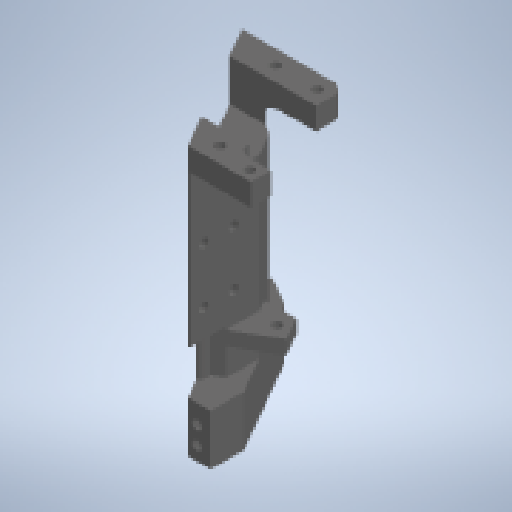
# Autodesk Inventor part: base_plate_towheel_front_left
Saved by Autodesk Inventor 2024.1 (Build 281209000, 209)
## iProperties
Created: 2025-02-03
Part Number: base_plate_towheel_front_left
Material: 一般
Document SubType Name: モデリング
Designer: hibik
Density: 1 g/cm^3
Appearance: 既定
Sheet Metal Rule: Default_mm
Author: hibik
Autodesk Inventor part; units mm, degrees
ref_plane "YZ Plane" through (0, 0, 0) normal (1, 0, 0) x (0, 1, 0)
ref_plane "XZ Plane" through (0, 0, 0) normal (0, 1, 0) x (-1, 0, 0)
ref_plane "XY Plane" through (0, 0, 0) normal (0, 0, 1) x (1, 0, 0)
sketch "スケッチ1" plane through (0, 0, 0) normal (0, 1, 0) x (-1, 0, 0)
  line L0 (75, 0) -> (105, -51.9615)
  line L1 (-75, 0) -> (-105, -51.9615)
  line L2 (0, -220.136) -> (0, 47.7586) projected
  line L3 (147, 0) -> (-147, 0) projected
  line L4 (37.5, -27) -> (-37.5, -27)
  line L5 (105, -51.9615) -> (30, -181.8653)
  line L6 (30, -181.8653) -> (-30, -181.8653)
  line L7 (-30, -181.8653) -> (-105, -51.9615)
  line L8 (75, 0) -> (-75, 0)
  line L9 (-25.3673, -135.8894) -> (-62.8673, -70.9375)
  line L10 (25.3673, -135.8894) -> (62.8673, -70.9375)
  line L11 (-37.5, -27) -> (-27.5, -27)
  line L12 (-27.5, -27) -> (-27.5, -39)
  line L13 (-27.5, -39) -> (-37.5, -39)
  line L14 (-37.5, -39) -> (-37.5, -27)
  line L15 (37.5, -27) -> (27.5, -27)
  line L16 (27.5, -27) -> (27.5, -39)
  line L17 (27.5, -39) -> (37.5, -39)
  line L18 (37.5, -39) -> (37.5, -27)
  line L19 (0, -77.9423) -> (44.1173, -103.4134) construction
  line L20 (0, -77.9423) -> (-44.1173, -103.4134) construction
  line L21 (-44.1173, -103.4134) -> (-67.5, -116.9134) construction
  line L22 (-57.8673, -79.5977) -> (-47.475, -73.5977)
  line L23 (-52.475, -64.9375) -> (-62.8673, -70.9375)
  line L24 (-62.8673, -70.9375) -> (-57.8673, -79.5977)
  line L25 (-47.475, -73.5977) -> (-52.475, -64.9375)
  line L26 (-25.3673, -135.8894) -> (-30.3673, -127.2291)
  line L27 (-19.975, -121.2291) -> (-14.975, -129.8894)
  line L28 (-14.975, -129.8894) -> (-25.3673, -135.8894)
  line L29 (-30.3673, -127.2291) -> (-19.975, -121.2291)
  line L30 (30.3673, -127.2291) -> (19.975, -121.2291)
  line L31 (14.975, -129.8894) -> (25.3673, -135.8894)
  line L32 (25.3673, -135.8894) -> (30.3673, -127.2291)
  line L33 (19.975, -121.2291) -> (14.975, -129.8894)
  line L34 (62.8673, -70.9375) -> (57.8673, -79.5977)
  line L35 (47.475, -73.5977) -> (52.475, -64.9375)
  line L36 (52.475, -64.9375) -> (62.8673, -70.9375)
  line L37 (57.8673, -79.5977) -> (47.475, -73.5977)
  line L38 (62.8673, -70.9375) -> (37.5, -27)
  line L39 (-37.5, -27) -> (-62.8673, -70.9375)
  line L40 (-25.3673, -135.8894) -> (25.3673, -135.8894)
  line L41 (-27.5, -39) -> (-47.475, -73.5977)
  point P0 (0, 0)
  point P1 (0, 0)
  point P2 (0, -27)
  dimension "d1" = 150
  dimension "d2" = 60
  dimension "d3" = 60
  dimension "d4" = 27
  dimension "d5" = 75
  dimension "d6" = 60
  dimension "d7" = 27
  dimension "d8" = 10
  dimension "d9" = 12
  dimension "d10" = 10
  dimension "d11" = 12
  dimension "d14" = 360
  constraints: 80 end point, 6 equal length, 6 parallel, 4 horizontal, 4 midpoint, 3 coincident, 3 perpendicular, 2 symmetric about line, 1 collinear, 1 horizontal alignment, 1 point on line, 1 vertical alignment, 50 other
  measures "d1" distance of L1.start L0.start
  measures "d2" angle of L3 L0
  measures "d3" angle of L1 L3
  measures "d4" distance between parallel lines of L3 L4
  measures "d5" distance of L4.start L4.end
  measures "d6" distance of L5.end L6.end
  measures "d7" distance between parallel lines of L7 L9
  measures "d8" distance of L12.end L13.end
  measures "d9" distance of L11.end L12.end
  measures "d10" distance of L17.end L16.end
  measures "d11" distance of L16.end L15.end
extrude "押し出し1" add sketch "スケッチ1" along normal blind 18.3 contours L12 L13 L14 L4 | L14 L13 L41 L25 L23 L39 | L23 L25 L22 L9
sketch "スケッチ2" plane through (27.5, 0, -27) normal (0, 0, 1) x (1, 0, 0)
  circle A0 centre (5, 11.5) radius 1.6 projected
  circle A1 centre (5, 5) radius 1.6 projected
  point P0 (-27.5, 0)
sketch "スケッチ3" plane through (27.5, 0, -27) normal (0, 0, 1) x (1, 0, 0)
  circle A0 centre (5, 11.5) radius 1.6 projected
  circle A1 centre (5, 5) radius 1.6 projected
  line L0 (8.2909, 11.5) -> (6.6454, 8.65)
  line L1 (6.6454, 8.65) -> (3.3546, 8.65)
  line L2 (3.3546, 8.65) -> (1.7091, 11.5)
  line L3 (1.7091, 11.5) -> (3.3546, 14.35)
  line L4 (3.3546, 14.35) -> (6.6454, 14.35)
  line L5 (6.6454, 14.35) -> (8.2909, 11.5)
  line L6 (6.6454, 7.85) -> (8.2909, 5)
  line L7 (8.2909, 5) -> (6.6454, 2.15)
  line L8 (6.6454, 2.15) -> (3.3546, 2.15)
  line L9 (3.3546, 2.15) -> (1.7091, 5)
  line L10 (1.7091, 5) -> (3.3546, 7.85)
  line L11 (3.3546, 7.85) -> (6.6454, 7.85)
  point P0 (-27.5, 0)
  dimension "d19" = 5.7
  constraints: 24 end point, 2 coincident, 2 horizontal, 1 parallel, 26 other
  measures "d19" distance from line of L0.end L4
extrude "押し出し2" cut sketch "スケッチ3" against normal blind 6 contours A0 | A1 | L0 L1 L2 L3 L4 L5 | L6 L7 L8 L9 L10 L11
extrude "押し出し3" add sketch "スケッチ3" against normal blind 3
sketch "スケッチ4" plane through (27.5, 0, -33) normal (0, 0, 1) x (1, 0, 0)
  line L0 (3.3546, 14.35) -> (6.6454, 14.35)
  line L1 (1.7091, 11.5) -> (3.3546, 14.35)
  line L2 (3.3546, 8.65) -> (1.7091, 11.5)
  line L3 (6.6454, 8.65) -> (3.3546, 8.65)
  line L4 (1.7091, 5) -> (3.3546, 7.85)
  line L5 (3.3546, 2.15) -> (1.7091, 5)
  line L6 (6.6454, 2.15) -> (3.3546, 2.15)
  line L7 (3.3546, 7.85) -> (6.6454, 7.85)
  line L8 (3.3546, 14.35) -> (6.6454, 14.35) projected
  line L9 (6.6454, 14.35) -> (42.8044, 14.35)
  line L10 (42.8044, 14.35) -> (42.8044, 8.65)
  line L11 (42.8044, 8.65) -> (6.6454, 8.65)
  line L12 (6.6454, 7.85) -> (42.8044, 7.85)
  line L13 (42.8044, 7.85) -> (42.8044, 2.15)
  line L14 (42.8044, 2.15) -> (6.6454, 2.15)
  line L15 (6.6454, 14.35) -> (3.3546, 14.35) projected
  line L16 (8.2909, 11.5) -> (6.6454, 14.35) projected
  line L17 (6.6454, 8.65) -> (8.2909, 11.5) projected
  line L18 (3.3546, 8.65) -> (6.6454, 8.65) projected
  line L19 (1.7091, 11.5) -> (3.3546, 8.65) projected
  line L20 (3.3546, 14.35) -> (1.7091, 11.5) projected
  circle A0 centre (5, 11.5) radius 1.6 projected
  line L21 (3.3546, 7.85) -> (1.7091, 5) projected
  line L22 (6.6454, 7.85) -> (3.3546, 7.85) projected
  line L23 (8.2909, 5) -> (6.6454, 7.85) projected
  line L24 (6.6454, 2.15) -> (8.2909, 5) projected
  line L25 (3.3546, 2.15) -> (6.6454, 2.15) projected
  line L26 (1.7091, 5) -> (3.3546, 2.15) projected
  circle A1 centre (5, 5) radius 1.6 projected
  line L27 (6.6454, 14.35) -> (3.3546, 14.35) projected
  line L28 (3.3546, 8.65) -> (6.6454, 8.65) projected
  line L29 (1.7091, 11.5) -> (3.3546, 8.65) projected
  line L30 (3.3546, 14.35) -> (1.7091, 11.5) projected
  line L31 (6.6454, 7.85) -> (3.3546, 7.85) projected
  line L32 (3.3546, 2.15) -> (6.6454, 2.15) projected
  line L33 (1.7091, 5) -> (3.3546, 2.15) projected
  line L34 (3.3546, 7.85) -> (1.7091, 5) projected
  point P0 (-27.5, 0)
  constraints: 28 end point, 2 horizontal, 2 parallel, 2 perpendicular, 2 point on line, 1 collinear
extrude "押し出し4" cut sketch "スケッチ4" along normal blind 3 contours L0 L16 L17 L3 L2 L1 | L9 L10 L11 L17 L16 | L4 L7 L23 L24 L6 L5 | L12 L13 L14 L24 L23 | A0 | A1
sketch "スケッチ5" plane through (62.8673, 0, -70.9375) normal (0.8660254, 0, 0.5) x (0.5, 0, -0.8660254)
  line L0 (-5.3923, 18.3) -> (-45.3423, 18.3) projected
  line L1 (-25.3673, 18.3) -> (-25.3673, 0)
  line L2 (-5.3923, 0) -> (-45.3423, 0) projected
  point P0 (-92.8673, 0)
  constraints: 2 end point, 2 midpoint
ref_plane "作業平面1" through (50.1837, 18.3, -48.9687) normal (-0.5, 0, 0.8660254) x (0, -1, 0)
mirror "ミラー1" about plane through (50.1837, 18.3, -48.9687) normal (-0.5, 0, 0.8660254) of "押し出し2", "押し出し3", "押し出し4"
sketch "スケッチ6" plane through (0, 0, 0) normal (0, -1, 0) x (1, 0, 0)
  line L0 (37.5, -27) -> (62.8673, -70.9375) projected
  circle A0 centre (40.9875, -45.0405) radius 1.6
  line L1 (42.7196, -48.0405) -> (39.2555, -48.0405)
  line L2 (39.2555, -48.0405) -> (37.5234, -45.0405)
  line L3 (37.5234, -45.0405) -> (39.2555, -42.0405)
  line L4 (39.2555, -42.0405) -> (42.7196, -42.0405)
  line L5 (42.7196, -42.0405) -> (44.4516, -45.0405)
  line L6 (44.4516, -45.0405) -> (42.7196, -48.0405)
  line L7 (50.1837, -48.9687) -> (37.4875, -56.2989)
  line L8 (47.475, -73.5977) -> (27.5, -39) projected
  line L9 (37.6966, -45.0405) -> (39.3421, -42.1905)
  line L10 (39.3421, -42.1905) -> (42.633, -42.1905)
  line L11 (42.633, -42.1905) -> (44.2784, -45.0405)
  line L12 (44.2784, -45.0405) -> (42.633, -47.8905)
  line L13 (42.633, -47.8905) -> (39.3421, -47.8905)
  line L14 (39.3421, -47.8905) -> (37.6966, -45.0405)
  point P0 (0, 0)
  dimension "d27" = 3.2
  dimension "d29" = 6
  dimension "d30" = 6
  dimension "d31" = 8
  dimension "d32" = 5.7
  constraints: 26 end point, 2 coincident, 2 midpoint, 2 parallel, 1 centre point, 26 other
  measures "d27" diameter of A0
  measures "d29" distance between parallel lines of L2 L5
  measures "d30" distance from line of L0 A0.centre
  measures "d31" distance from line of L7 A0.centre
  measures "d32" distance between parallel lines of L14 L11
extrude "押し出し5" cut sketch "スケッチ6" against normal through all contours A0 | L9 L10 L11 L12 L13 L14
extrude "押し出し7" add sketch "スケッチ6" against normal blind 3 contours L9 L10 L11 L12 L13 L14
mirror "ミラー2" about plane through (50.1837, 18.3, -48.9687) normal (-0.5, 0, 0.8660254) of "押し出し5", "押し出し7"
sketch "スケッチ10" plane through (0, 0, 0) normal (0, -1, 0) x (1, 0, 0)
  line L0 (75, 0) -> (105, -51.9615)
  line L1 (75, 0) -> (81.3804, 3.6837)
  line L2 (37.5, -27) -> (62.8673, -70.9375) projected
  line L3 (50.1837, -48.9687) -> (90, -25.9808)
  line L4 (-21, 0) -> (126, 0) projected
  line L5 (75, 0) -> (35, 0)
  line L6 (45, 0) -> (45, -18)
  line L7 (45, -18) -> (35, -23.7735)
  line L8 (35, 0) -> (35, -23.7735)
  line L9 (35, -23.7735) -> (49.7058, -49.2446)
  line L10 (105, -51.9615) -> (75, 0)
  line L11 (85, -86.6025) -> (64.4115, -74.7158)
  line L12 (64.4115, -74.7158) -> (49.7058, -49.2446)
  line L13 (85, -86.6025) -> (105, -51.9615)
  line L14 (62.8673, -70.9375) -> (57.8673, -79.5977) projected
  line L15 (61.9714, -72.4893) -> (35.6987, -26.9836)
  line L16 (27.5, -27) -> (37.5, -27) projected
  point P0 (0, 0)
  point P1 (35.7081, -27)
  dimension "d47" = 60
  dimension "d48" = 40
  dimension "d49" = 18
  dimension "d50" = 30
  dimension "d51" = 60
  dimension "d63" = 1
  constraints: 28 end point, 5 perpendicular, 5 point on line, 4 symmetric about line, 2 midpoint, 2 parallel
  measures "d47" distance from line of L0.end L1
  measures "d48" distance of L5.end L0.start
  measures "d49" distance of L6.start L6.end
  measures "d50" distance of L0.start L6.start
  measures "d51" angle of L6 L7
  measures "d63" distance between parallel lines of L12 L15
sketch "スケッチ8" plane through (0, 18.3, 0) normal (0, 1, 0) x (1, 0, 0)
  line L0 (47.475, 73.5977) -> (27.5, 39) projected
  line L1 (47.3421, 61.7469) -> (50.633, 61.7469) projected
  line L2 (50.633, 61.7469) -> (52.2784, 58.8969) projected
  line L3 (52.2784, 58.8969) -> (50.633, 56.0469) projected
  line L4 (50.633, 56.0469) -> (47.3421, 56.0469) projected
  line L5 (47.3421, 56.0469) -> (45.6966, 58.8969) projected
  line L6 (45.6966, 58.8969) -> (47.3421, 61.7469) projected
  line L7 (42.633, 47.8905) -> (44.2784, 45.0405) projected
  line L8 (44.2784, 45.0405) -> (42.633, 42.1905) projected
  line L9 (42.633, 42.1905) -> (39.3421, 42.1905) projected
  line L10 (39.3421, 42.1905) -> (37.6966, 45.0405) projected
  line L11 (37.6966, 45.0405) -> (39.3421, 47.8905) projected
  line L12 (39.3421, 47.8905) -> (42.633, 47.8905) projected
  line L13 (57.8673, 79.5977) -> (47.475, 73.5977) projected
  line L14 (47.475, 73.5977) -> (27.5, 39) projected
  line L15 (27.5, 39) -> (27.5, 27) projected
  line L16 (27.5, 27) -> (37.5, 27) projected
  line L17 (37.5, 27) -> (62.8673, 70.9375) projected
  line L18 (62.8673, 70.9375) -> (57.8673, 79.5977) projected
  line L19 (42.633, 47.8905) -> (47.8291, 44.8905)
  line L20 (39.3421, 42.1905) -> (44.5382, 39.1905)
  line L21 (47.3421, 56.0469) -> (52.5382, 53.0469)
  line L22 (50.633, 61.7469) -> (55.8291, 58.7469)
  line L23 (37.5, 27) -> (62.8673, 70.9375) projected
  point P0 (0, 0)
  constraints: 8 end point, 4 perpendicular, 4 point on line
extrude "押し出し9" cut sketch "スケッチ8" against normal up to surface (15.3 mm away) contours L17 L21 L4 L3 L2 L22 | L20 L9 L8 L7 L19 L17
sketch "スケッチ11" plane through (0, 18.3, 0) normal (0, 1, 0) x (1, 0, 0)
  line L0 (52.5382, 53.0469) -> (47.3421, 56.0469) projected
  line L1 (47.3421, 56.0469) -> (45.6966, 58.8969) projected
  line L2 (45.6966, 58.8969) -> (47.3421, 61.7469) projected
  line L3 (47.3421, 61.7469) -> (50.633, 61.7469) projected
  line L4 (50.633, 61.7469) -> (55.8291, 58.7469) projected
  line L5 (55.8291, 58.7469) -> (62.8673, 70.9375) projected
  line L6 (62.8673, 70.9375) -> (57.8673, 79.5977) projected
  line L7 (57.8673, 79.5977) -> (47.475, 73.5977) projected
  line L8 (47.475, 73.5977) -> (27.5, 39) projected
  line L9 (27.5, 39) -> (27.5, 27) projected
  line L10 (27.5, 27) -> (37.5, 27) projected
  line L11 (37.5, 27) -> (44.5382, 39.1905) projected
  line L12 (44.5382, 39.1905) -> (39.3421, 42.1905) projected
  line L13 (39.3421, 42.1905) -> (37.6966, 45.0405) projected
  line L14 (37.6966, 45.0405) -> (39.3421, 47.8905) projected
  line L15 (39.3421, 47.8905) -> (42.633, 47.8905) projected
  line L16 (42.633, 47.8905) -> (47.8291, 44.8905) projected
  line L17 (47.8291, 44.8905) -> (52.5382, 53.0469) projected
  line L18 (38.5, 27) -> (38.5, 38)
  line L19 (38.5, 38) -> (29.817, 43.0131)
  line L20 (27.5, 27) -> (37.5, 27) projected
  line L21 (47.475, 73.5977) -> (27.5, 39) projected
  line L22 (50.1837, 48.9687) -> (37.4875, 56.2989)
  line L23 (63.3673, 70.0715) -> (53.841, 64.5715)
  line L24 (53.841, 64.5715) -> (45.158, 69.5846)
  line L25 (47.8291, 44.8905) -> (44.5382, 39.1905) projected
  line L26 (55.8291, 58.7469) -> (52.5382, 53.0469) projected
  point P0 (0, 0)
  point P1 (61.8673, 69.2054)
  point P2 (38.5, 28.7321)
  dimension "d52" = 1
  dimension "d53" = 11
  constraints: 10 end point, 3 perpendicular, 3 symmetric about line, 2 midpoint, 2 point on line
  measures "d52" distance from line of L10.end L18
  measures "d53" distance of L18.start L18.end
extrude "押し出し11" add sketch "スケッチ11" along normal blind 78.7 contours L17 L22 L8 L24 L23 L5 L4 L3 L2 L1 L0 | L0 L1 L2 L3 L4 L26 | L17 L16 L15 L14 L13 L12 L11 L18 L19 L8 L22 | L25 L12 L13 L14 L15 L16
fillet "フィレット1" radius 2 2 edges at (38.5, 57.65, -28.7321) (61.8673, 57.65, -69.2054)
sketch "スケッチ13" plane through (0, 97, 0) normal (0, 1, 0) x (1, 0, 0)
  line L0 (85, 86.6025) -> (64.4115, 74.7158) projected
  line L1 (35, 0) -> (35, 23.7735) projected
  arc A0 (58.1353, 62.7413) -> (55.4032, 65.4734) centre (56.4032, 63.7413) ccw projected
  line L2 (55.4032, 65.4734) -> (53.841, 64.5715) projected
  line L3 (53.841, 64.5715) -> (45.158, 69.5846) projected
  line L4 (45.158, 69.5846) -> (29.817, 43.0131) projected
  line L5 (29.817, 43.0131) -> (38.5, 38) projected
  line L6 (38.5, 38) -> (38.5, 36.1962) projected
  arc A1 (38.5, 36.1962) -> (42.2321, 35.1962) centre (40.5, 36.1962) ccw projected
  line L7 (35, 23.7735) -> (35, 57.735)
  line L8 (35, 57.735) -> (64.4115, 74.7158)
  line L9 (38.5, 38) -> (29.817, 43.0131) projected
  line L10 (29.817, 43.0131) -> (27.5, 39) projected
  line L11 (27.5, 39) -> (27.5, 27) projected
  line L12 (27.5, 27) -> (37.5, 27) projected
  line L13 (37.5, 27) -> (42.2321, 35.1962) projected
  arc A2 (38.5, 36.1962) -> (42.2321, 35.1962) centre (40.5, 36.1962) ccw projected
  line L14 (38.5, 36.1962) -> (38.5, 38) projected
  line L15 (45.158, 69.5846) -> (53.841, 64.5715) projected
  line L16 (53.841, 64.5715) -> (55.4032, 65.4734) projected
  arc A3 (58.1353, 62.7413) -> (55.4032, 65.4734) centre (56.4032, 63.7413) ccw projected
  line L17 (58.1353, 62.7413) -> (62.8673, 70.9375) projected
  line L18 (62.8673, 70.9375) -> (57.8673, 79.5977) projected
  line L19 (57.8673, 79.5977) -> (47.475, 73.5977) projected
  line L20 (47.475, 73.5977) -> (45.158, 69.5846) projected
  line L21 (42.2321, 35.1962) -> (58.1353, 62.7413) projected
  point P0 (0, 0)
  point P1 (61.6173, 73.1025)
  point P2 (50.341, 66.5922)
  point P3 (39.975, 60.6073)
  point P4 (35, 51.9904)
  point P5 (35, 27)
  point P6 (35, 40.0207)
  constraints: 4 end point, 1 collinear, 1 vertical
extrude "押し出し13" add sketch "スケッチ13" against normal blind 62.7 contours A0 L2 L3 L8 L18 L17 | L13 L12 L7 L5 L6 A1 | L4 L7 L8
extrude "押し出し14" cut sketch "スケッチ13" against normal up to surface (78.7 mm away) contours L8 L4 L3 | L5 L4 L7
extrude "押し出し15" cut sketch "スケッチ10" against normal through all contours L2 L14 L12 L9 L16 | L9 L12 L14 L15 L16
sketch "スケッチ14" plane through (0, 97, 0) normal (0, 1, 0) x (1, 0, 0)
  circle A0 centre (75, 50.5) radius 8.0371 projected
  circle A1 centre (75, 50.5) radius 12
  line L0 (75, 62.5) -> (35, 62.5)
  line L1 (35, 62.5) -> (35, 38.5)
  line L2 (35, 38.5) -> (75, 38.5)
  line L3 (75, 38.5) -> (75, 62.5)
  line L4 (35, 57.735) -> (35, 27) projected
  point P0 (0, 0)
  dimension "d66" = 24
  constraints: 8 end point, 3 horizontal, 2 parallel, 1 coincident, 1 collinear, 1 perpendicular, 3 other
extrude "押し出し16" cut sketch "スケッチ14" against normal blind 15 contours A1 L2 L1 L0
sketch "スケッチ15" plane through (61.6173, 34.3, -73.1025) normal (-0.5, 0, -0.8660254) x (-0.8660254, 0, 0.5)
  circle A0 centre (5, 10) radius 1.6
  circle A1 centre (15.735, 10) radius 1.6
  line L0 (0, 62.7) -> (0, 0) projected
  line L1 (30.735, 47.7) -> (30.735, 0) projected
  line L2 (13.0207, 0) -> (0, 0) projected
  circle A2 centre (15.735, 30) radius 1.6
  circle A3 centre (5, 30) radius 1.6
  circle A4 centre (15.735, 50) radius 1.6
  circle A5 centre (5, 50) radius 1.6
  point P0 (89.9134, -34.3)
  dimension "d69" = 3.2
  dimension "d71" = 5
  dimension "d72" = 15
  dimension "d73" = 10
  dimension "d76" = 20
  constraints: 6 centre point, 1 equal radius, 1 horizontal alignment, 1 vertical, 8 other
  measures "d69" diameter of A0
  measures "d71" distance from line of L0 A0.centre
  measures "d72" distance from line of L1 A1.centre
  measures "d73" distance from line of L2 A0.centre
  measures "d76" distance of A1.centre A2.centre
extrude "押し出し17" cut sketch "スケッチ15" against normal through all contours A0 | A1 | A2 | A3
ref_plane "作業平面3" through (71.6173, 34.3, -55.782) normal (-0.5, 0, -0.8660254) x (-0.8660254, 0, 0.5)
sketch "スケッチ17" plane through (71.6173, 34.3, -55.782) normal (-0.5, 0, -0.8660254) x (-0.8660254, 0, 0.5)
  circle A0 centre (5, 10) radius 1.6 projected
  circle A1 centre (15.735, 10) radius 1.6 projected
  circle A2 centre (5, 30) radius 1.6 projected
  circle A3 centre (15.735, 30) radius 1.6 projected
  line L0 (30.735, 47.7) -> (21.2051, 47.7) projected
  line L1 (21.2051, 47.7) -> (21.2051, 62.7) projected
  line L2 (0, 62.7) -> (21.2051, 62.7) projected
  line L3 (0, 62.7) -> (0, 0) projected
  line L4 (13.0207, 0) -> (0, 0) projected
  line L5 (13.0207, -16) -> (13.0207, 0) projected
  line L6 (13.0207, -16) -> (24.9904, -16) projected
  line L7 (24.9904, 0) -> (24.9904, -16) projected
  line L8 (30.735, 0) -> (24.9904, 0) projected
  line L9 (30.735, 47.7) -> (30.735, 0) projected
  line L10 (2.9233, 48.4535) -> (1.2201, 51.4035)
  line L11 (1.2201, 51.4035) -> (2.9233, 54.3535)
  line L12 (2.9233, 54.3535) -> (6.3297, 54.3535)
  line L13 (6.3297, 54.3535) -> (8.0329, 51.4035)
  line L14 (8.0329, 51.4035) -> (6.3297, 48.4535)
  line L15 (6.3297, 48.4535) -> (2.9233, 48.4535)
  line L16 (14.0318, 27.05) -> (12.3287, 30)
  line L17 (12.3287, 30) -> (14.0318, 32.95)
  line L18 (14.0318, 32.95) -> (17.4382, 32.95)
  line L19 (17.4382, 32.95) -> (19.1414, 30)
  line L20 (19.1414, 30) -> (17.4382, 27.05)
  line L21 (17.4382, 27.05) -> (14.0318, 27.05)
  line L22 (3.2968, 27.05) -> (1.5936, 30)
  line L23 (1.5936, 30) -> (3.2968, 32.95)
  line L24 (3.2968, 32.95) -> (6.7032, 32.95)
  line L25 (6.7032, 32.95) -> (8.4064, 30)
  line L26 (8.4064, 30) -> (6.7032, 27.05)
  line L27 (6.7032, 27.05) -> (3.2968, 27.05)
  line L28 (14.0318, 7.05) -> (12.3287, 10)
  line L29 (12.3287, 10) -> (14.0318, 12.95)
  line L30 (14.0318, 12.95) -> (17.4382, 12.95)
  line L31 (17.4382, 12.95) -> (19.1414, 10)
  line L32 (19.1414, 10) -> (17.4382, 7.05)
  line L33 (17.4382, 7.05) -> (14.0318, 7.05)
  line L34 (6.7032, 7.05) -> (3.2968, 7.05)
  line L35 (3.2968, 7.05) -> (1.5936, 10)
  line L36 (1.5936, 10) -> (3.2968, 12.95)
  line L37 (3.2968, 12.95) -> (6.7032, 12.95)
  line L38 (6.7032, 12.95) -> (8.4064, 10)
  line L39 (8.4064, 10) -> (6.7032, 7.05)
  point P0 (89.9134, -34.3)
  point P1 (4.6265, 51.4035)
  point P2 (15.735, 30)
  point P3 (5, 30)
  point P4 (15.735, 10)
  point P5 (5, 10)
  dimension "d84" = 5.9
  constraints: 60 end point, 4 coincident, 4 equal length, 4 horizontal, 1 point on line, 65 other
  measures "d84" distance between parallel lines of L33 L30
extrude "押し出し18" cut sketch "スケッチ17" along normal blind 18 contours A0 | A1 | A2 | A3 | L16 L17 L18 L19 L20 L21 | L22 L23 L24 L25 L26 L27 | L28 L29 L30 L31 L32 L33 | L34 L35 L36 L37 L38 L39
ref_plane "作業平面4" through (35, 97, -57.735) normal (0.5, 0, -0.8660254) x (0, -1, 0)
mirror "ミラー4" about plane through (35, 97, -57.735) normal (0.5, 0, -0.8660254) of "押し出し17", "押し出し18"
sketch "スケッチ20" plane through (0, 97, 0) normal (0, 1, 0) x (1, 0, 0)
  line L0 (42.3476, 38.5) -> (25, 38.5)
  line L1 (25, 38.5) -> (25, 27)
  line L2 (25, 27) -> (42.3476, 27)
  line L3 (42.3476, 27) -> (42.3476, 38.5) construction
  line L4 (61.9714, 62.5) -> (25, 62.5)
  line L5 (25, 62.5) -> (25, 73.1025)
  line L6 (25, 73.1025) -> (61.9714, 73.1025)
  line L7 (61.9714, 73.1025) -> (61.9714, 62.5) construction
  line L8 (42.3476, 38.5) -> (35, 38.5) projected
  line L9 (43.2532, 62.5) -> (56.2041, 62.5) projected
  line L10 (35.7081, 27) -> (42.3476, 38.5) projected
  line L11 (35, 38.5) -> (35, 27) projected
  line L12 (56.2041, 62.5) -> (61.9714, 72.4893) projected
  line L13 (61.9714, 72.4893) -> (61.6173, 73.1025) projected
  point P0 (0, 0)
  dimension "d88" = 25
  constraints: 16 end point, 4 parallel, 4 point on line, 3 collinear, 2 horizontal, 2 perpendicular
  measures "d88" distance from line of L5 point (0, 0)
extrude "押し出し19" add sketch "スケッチ20" against normal blind 8
fillet "フィレット2" radius 3 1 edges at (52.4352, 89, -67.8013)
sketch "スケッチ21" plane through (0, 97, 0) normal (0, 1, 0) x (1, 0, 0)
  circle A0 centre (30, 32.75) radius 1.6
  circle A1 centre (30, 67.8013) radius 1.6
  circle A2 centre (45, 67.8013) radius 1.6
  line L0 (25, 38.5) -> (25, 27) projected
  line L1 (25, 73.1025) -> (25, 62.5) projected
  point P0 (0, 0)
  point P1 (25, 32.75)
  point P2 (25, 67.8013)
  dimension "d92" = 3.2
  dimension "d94" = 5
  dimension "d95" = 15
  constraints: 3 centre point, 3 horizontal alignment, 2 equal radius, 2 midpoint, 1 vertical alignment
  measures "d92" diameter of A0
  measures "d94" distance from line of L0 A0.centre
  measures "d95" distance of A1.centre A2.centre
extrude "押し出し20" cut sketch "スケッチ21" against normal blind 15
ref_plane "作業平面5" through (0, 82, 0) normal (0, 1, 0) x (1, 0, 0)
sketch "スケッチ22" plane through (0, 82, 0) normal (0, 1, 0) x (1, 0, 0)
  circle A0 centre (30, 32.75) radius 1.6 projected
  circle A1 centre (30, 67.8013) radius 1.6 projected
  circle A2 centre (45, 67.8013) radius 1.6 projected
  line L0 (28.3546, 35.6) -> (31.6454, 35.6)
  line L1 (31.6454, 35.6) -> (33.2909, 32.75)
  line L2 (33.2909, 32.75) -> (31.6454, 29.9)
  line L3 (31.6454, 29.9) -> (28.3546, 29.9)
  line L4 (28.3546, 29.9) -> (26.7091, 32.75)
  line L5 (26.7091, 32.75) -> (28.3546, 35.6)
  line L6 (43.3546, 70.6513) -> (46.6454, 70.6513)
  line L7 (46.6454, 70.6513) -> (48.2909, 67.8013)
  line L8 (48.2909, 67.8013) -> (46.6454, 64.9513)
  line L9 (46.6454, 64.9513) -> (43.3546, 64.9513)
  line L10 (43.3546, 64.9513) -> (41.7091, 67.8013)
  line L11 (41.7091, 67.8013) -> (43.3546, 70.6513)
  line L12 (28.3546, 70.6513) -> (31.6454, 70.6513)
  line L13 (31.6454, 70.6513) -> (33.2909, 67.8013)
  line L14 (33.2909, 67.8013) -> (31.6454, 64.9513)
  line L15 (31.6454, 64.9513) -> (28.3546, 64.9513)
  line L16 (28.3546, 64.9513) -> (26.7091, 67.8013)
  line L17 (26.7091, 67.8013) -> (28.3546, 70.6513)
  point P0 (0, 0)
  dimension "d99" = 5.7
  constraints: 36 end point, 4 coincident, 2 equal length, 2 horizontal, 1 horizontal alignment, 39 other
  measures "d99" distance between parallel lines of L0 L3
extrude "押し出し21" cut sketch "スケッチ22" along normal blind 13 contours A2 | L6 L7 L8 L9 L10 L11
mirror "ミラー5" about plane through (0, 0, 0) normal (1, 0, 0) remove original yes
ref_plane "作業平面6" through (0, 33.3, -87.9447) normal (0, -1, 0) x (1, 0, 0)
sketch "スケッチ23" plane through (0, 33.3, -87.9447) normal (0, -1, 0) x (1, 0, 0)
  circle A0 centre (-37.2789, 20.0072) radius 1.6 projected
  circle A1 centre (-27.3038, 37.2844) radius 1.6 projected
  line L0 (-35, 60.9447) -> (-35, 47.924) projected
  line L1 (-35, 35.9543) -> (-35, 47.924) projected
  line L2 (-35, 35.9543) -> (-35, 30.2097) projected
  line L3 (-35, 49.4447) -> (-35, 30.2097) projected
  line L4 (-35, 43.6097) -> (-35, 46.8097) projected
  line L5 (-35, 54.3447) -> (-35, 57.5447) projected
  line L6 (-35, 43.6097) -> (-35, 46.8097) projected
  line L7 (-35, 54.3447) -> (-35, 57.5447) projected
  line L8 (-61.6173, 14.8422) -> (-43.2532, 25.4447) projected
  line L9 (-35, 30.2097) -> (-43.2532, 25.4447) projected
  line L10 (-35, 30.2097) -> (-39.975, 27.3373) projected
  line L11 (-50.341, 21.3525) -> (-39.975, 27.3373) projected
  line L12 (-50.341, 21.3525) -> (-61.6173, 14.8422) projected
  line L13 (-49.376, 21.9097) -> (-46.6047, 23.5097) projected
  line L14 (-58.6728, 16.5422) -> (-55.9015, 18.1422) projected
  line L15 (-49.376, 21.9097) -> (-46.6047, 23.5097) projected
  line L16 (-58.6728, 16.5422) -> (-55.9015, 18.1422) projected
  line L17 (-35, 47.924) -> (-21.1567, 39.9316)
  line L18 (-21.1567, 39.9316) -> (-36.4978, 13.3601)
  line L19 (-36.4978, 13.3601) -> (-50.341, 21.3525)
  line L20 (-54.4852, 28.4218) -> (-51.1943, 34.1218) projected
  line L21 (-51.1943, 34.1218) -> (-54.4852, 28.4218) projected
  line L22 (-46.4852, 42.2782) -> (-43.1943, 47.9782) projected
  line L23 (-43.1943, 47.9782) -> (-46.4852, 42.2782) projected
  line L24 (-53.8701, 29.4872) -> (-51.9034, 32.8936) projected
  line L25 (-54.8534, 27.7841) -> (-53.8701, 29.4872) projected
  line L26 (-53.8701, 29.4872) -> (-54.8534, 27.7841) projected
  line L27 (-51.9034, 32.8936) -> (-53.8701, 29.4872) projected
  line L28 (-50.9201, 34.5968) -> (-51.9034, 32.8936) projected
  line L29 (-51.9034, 32.8936) -> (-50.9201, 34.5968) projected
  line L30 (-53.8701, 29.4872) -> (-51.9034, 32.8936) projected
  line L31 (-54.8534, 27.7841) -> (-53.8701, 29.4872) projected
  line L32 (-53.8701, 29.4872) -> (-54.8534, 27.7841) projected
  line L33 (-51.9034, 32.8936) -> (-53.8701, 29.4872) projected
  line L34 (-50.9201, 34.5968) -> (-51.9034, 32.8936) projected
  line L35 (-51.9034, 32.8936) -> (-50.9201, 34.5968) projected
  line L36 (-60.068, 18.7522) -> (-60.6795, 17.693) projected
  line L37 (-58.1013, 22.1586) -> (-60.068, 18.7522) projected
  line L38 (-57.118, 23.8618) -> (-58.1013, 22.1586) projected
  line L39 (-58.1013, 22.1586) -> (-57.118, 23.8618) projected
  line L40 (-60.068, 18.7522) -> (-58.1013, 22.1586) projected
  line L41 (-60.6795, 17.693) -> (-60.068, 18.7522) projected
  line L42 (-60.068, 18.7522) -> (-60.6795, 17.693) projected
  line L43 (-58.1013, 22.1586) -> (-60.068, 18.7522) projected
  line L44 (-57.118, 23.8618) -> (-58.1013, 22.1586) projected
  line L45 (-58.1013, 22.1586) -> (-57.118, 23.8618) projected
  line L46 (-60.068, 18.7522) -> (-58.1013, 22.1586) projected
  line L47 (-60.6795, 17.693) -> (-60.068, 18.7522) projected
  line L48 (-45.7761, 43.5065) -> (-43.8094, 46.9128) projected
  line L49 (-46.7594, 41.8033) -> (-45.7761, 43.5065) projected
  line L50 (-45.7761, 43.5065) -> (-46.7594, 41.8033) projected
  line L51 (-43.8094, 46.9128) -> (-45.7761, 43.5065) projected
  line L52 (-42.8261, 48.616) -> (-43.8094, 46.9128) projected
  line L53 (-43.8094, 46.9128) -> (-42.8261, 48.616) projected
  line L54 (-39.5782, 54.2415) -> (-37.6115, 57.6479) projected
  line L55 (-40.5615, 52.5383) -> (-39.5782, 54.2415) projected
  line L56 (-39.5782, 54.2415) -> (-40.5615, 52.5383) projected
  line L57 (-37.6115, 57.6479) -> (-39.5782, 54.2415) projected
  line L58 (-37, 58.7071) -> (-37.6115, 57.6479) projected
  line L59 (-37.6115, 57.6479) -> (-37, 58.7071) projected
  line L60 (-45.7761, 43.5065) -> (-43.8094, 46.9128) projected
  line L61 (-46.7594, 41.8033) -> (-45.7761, 43.5065) projected
  line L62 (-45.7761, 43.5065) -> (-46.7594, 41.8033) projected
  line L63 (-43.8094, 46.9128) -> (-45.7761, 43.5065) projected
  line L64 (-42.8261, 48.616) -> (-43.8094, 46.9128) projected
  line L65 (-43.8094, 46.9128) -> (-42.8261, 48.616) projected
  line L66 (-40.5615, 52.5383) -> (-39.5782, 54.2415) projected
  line L67 (-39.5782, 54.2415) -> (-40.5615, 52.5383) projected
  line L68 (-37.6115, 57.6479) -> (-39.5782, 54.2415) projected
  line L69 (-37, 58.7071) -> (-37.6115, 57.6479) projected
  line L70 (-37.6115, 57.6479) -> (-37, 58.7071) projected
  line L71 (-39.5782, 54.2415) -> (-37.6115, 57.6479) projected
  line L72 (-56.2041, 25.4447) -> (-61.9714, 15.4554) projected
  line L73 (-61.9714, 15.4554) -> (-57.7659, 22.7395) projected
  line L74 (-57.7659, 22.7395) -> (-61.9714, 15.4554) projected
  line L75 (-61.9714, 15.4554) -> (-35.7081, 60.9447) projected
  line L76 (-35.7081, 60.9447) -> (-39.9136, 53.6606) projected
  line L77 (-39.9136, 53.6606) -> (-35.7081, 60.9447) projected
  line L78 (-35.7081, 60.9447) -> (-42.3476, 49.4447) projected
  line L79 (-56.2041, 25.4447) -> (-42.3476, 49.4447) projected
  line L80 (-35, 30.2097) -> (-28.8273, 26.6458)
  line L81 (-35, 35.9543) -> (-39.975, 27.3373) projected
  line L82 (-35, 30.2097) -> (-37.4875, 31.6458)
  line L83 (-37.4875, 31.6458) -> (-25.9405, 31.6458)
  line L84 (-60.2393, 18.4554) -> (-58.5073, 21.4554) projected
  line L85 (-58.5073, 21.4554) -> (-60.2393, 18.4554) projected
  line L86 (-60.2393, 18.4554) -> (-58.5073, 21.4554) projected
  line L87 (-58.5073, 21.4554) -> (-60.2393, 18.4554) projected
  line L88 (-37.4402, 57.9447) -> (-39.1722, 54.9447) projected
  line L89 (-39.1722, 54.9447) -> (-37.4402, 57.9447) projected
  line L90 (-37.4402, 57.9447) -> (-39.1722, 54.9447) projected
  line L91 (-39.1722, 54.9447) -> (-37.4402, 57.9447) projected
  line L92 (-35, 60.9447) -> (-35, 49.4447) projected
  point P0 (0, 87.9447)
  point P1 (-43.2532, 25.4447)
  point P2 (-50.341, 21.3525)
  point P3 (-39.975, 27.3373)
  dimension "d102" = 4
  constraints: 12 end point, 3 perpendicular, 2 midpoint, 1 horizontal, 1 parallel, 1 point on line
  measures "d102" distance from line of L18 A1.centre
extrude "押し出し22" add sketch "スケッチ23" along normal blind 5 contours L1 L17 L18 L83 L2 | L2 L83 L81
sketch "スケッチ25" plane through (0, 28.3, -87.9447) normal (0, -1, 0) x (1, 0, 0)
  line L0 (-35, 43.6097) -> (-35, 46.8097) projected
  line L1 (-35, 49.4447) -> (-35, 60.9447) projected
  line L2 (-21.1567, 39.9316) -> (-35, 47.924) projected
  line L3 (-35, 35.9543) -> (-35, 47.924) projected
  line L4 (-37.4875, 31.6458) -> (-35, 35.9543) projected
  line L5 (-25.9405, 31.6458) -> (-21.1567, 39.9316) projected
  circle A0 centre (-27.3038, 37.2844) radius 1.6 projected
  line L6 (-28.9493, 34.4344) -> (-30.5947, 37.2844)
  line L7 (-30.5947, 37.2844) -> (-28.9493, 40.1344)
  line L8 (-28.9493, 40.1344) -> (-25.6584, 40.1344)
  line L9 (-25.6584, 40.1344) -> (-24.013, 37.2844)
  line L10 (-24.013, 37.2844) -> (-25.6584, 34.4344)
  line L11 (-25.6584, 34.4344) -> (-28.9493, 34.4344)
  line L12 (-38.9243, 22.8572) -> (-35.6334, 22.8572)
  line L13 (-35.6334, 22.8572) -> (-33.988, 20.0072)
  line L14 (-33.988, 20.0072) -> (-35.6334, 17.1572)
  line L15 (-35.6334, 17.1572) -> (-38.9243, 17.1572)
  line L16 (-38.9243, 17.1572) -> (-40.5698, 20.0072)
  line L17 (-40.5698, 20.0072) -> (-38.9243, 22.8572)
  line L18 (-37.4875, 31.6458) -> (-25.9405, 31.6458) projected
  point P0 (0, 87.9447)
  point P1 (-27.3038, 37.2844)
  point P2 (-37.2789, 20.0072)
  dimension "d105" = 5.7
  constraints: 24 end point, 2 parallel, 1 coincident, 1 collinear, 26 other
  measures "d105" distance between parallel lines of L7 L10
extrude "押し出し23" cut sketch "スケッチ25" against normal blind 2 contours A0 | L6 L7 L8 L9 L10 L11 | L12 L13 L14 L15 L16 L17
sketch "スケッチ26" plane through (-37, 63.1846, -29.2376) normal (-1, 0, 0) x (0, 0, 1)
  circle A0 centre (-13.4974, 1.1154) radius 1.6 projected
  circle A1 centre (-2.7624, 1.1154) radius 1.6 projected
  circle A2 centre (-2.7624, -18.8846) radius 1.6 projected
  circle A3 centre (-13.4974, -18.8846) radius 1.6 projected
  circle A4 centre (-13.4974, 1.1154) radius 4
  circle A5 centre (-2.7624, 1.1154) radius 4
  circle A6 centre (-2.7624, -18.8846) radius 4
  circle A7 centre (-13.4974, -18.8846) radius 4
  point P0 (29.2376, -63.1846)
  dimension "d108" = 8
  constraints: 4 centre point, 4 coincident, 3 equal radius
  measures "d108" diameter of A5
extrude "押し出し24" cut sketch "スケッチ26" along normal through all contours A0 | A1 | A2 | A3 | A4 | A5 | A6 | A7
sketch "スケッチ28" plane through (-42.633, 18.3, -47.8905) normal (0, -1, 0) x (1, 0, 0)
  line L0 (-11.8522, -11.6323) -> (-8.5613, -5.9323) projected
  line L1 (-8, -13.8564) -> (-11.8522, -11.6323) projected
  line L2 (-4.7091, -13.8564) -> (-8, -13.8564) projected
  line L3 (-3.0637, -11.0064) -> (-4.7091, -13.8564) projected
  line L4 (-4.7091, -8.1564) -> (-3.0637, -11.0064) projected
  line L5 (-8.5613, -5.9323) -> (-4.7091, -8.1564) projected
  line L6 (-3.8522, 2.2241) -> (-0.5613, 7.9241) projected
  line L7 (0, 0) -> (-3.8522, 2.2241) projected
  line L8 (3.2909, 0) -> (0, 0) projected
  line L9 (4.9363, 2.85) -> (3.2909, 0) projected
  line L10 (3.2909, 5.7) -> (4.9363, 2.85) projected
  line L11 (-0.5613, 7.9241) -> (3.2909, 5.7) projected
  point P0 (42.633, 47.8905)
extrude "押し出し25" add sketch "スケッチ28" along normal blind 12.3
sketch "スケッチ29" plane through (-58.5073, 8.65, -66.4893) normal (-0.8660254, 0, -0.5) x (-0.5, 0, 0.8660254)
  line L0 (0, 5.7) -> (0, 0) projected
  line L1 (-8.3177, 5.7) -> (0, 5.7) projected
  line L2 (-9.9631, 2.85) -> (-8.3177, 5.7) projected
  line L3 (-8.3177, 0) -> (-9.9631, 2.85) projected
  line L4 (-8.3177, 0) -> (0, 0) projected
  line L5 (0, -0.8) -> (0, -6.5) projected
  line L6 (-8.3177, -0.8) -> (0, -0.8) projected
  line L7 (-9.9631, -3.65) -> (-8.3177, -0.8) projected
  line L8 (-8.3177, -6.5) -> (-9.9631, -3.65) projected
  line L9 (-8.3177, -6.5) -> (0, -6.5) projected
  circle A0 centre (-6.6722, -3.65) radius 1.6 projected
  circle A1 centre (-6.6722, 2.85) radius 1.6 projected
  line L10 (-8.3177, 5.7) -> (-5.0268, 5.7)
  line L11 (-5.0268, 5.7) -> (-3.3813, 2.85)
  line L12 (-3.3813, 2.85) -> (-5.0268, 0)
  line L13 (-5.0268, 0) -> (-8.3177, 0)
  line L14 (-8.3177, 0) -> (-9.9631, 2.85)
  line L15 (-9.9631, 2.85) -> (-8.3177, 5.7)
  line L16 (-9.9631, -3.65) -> (-8.3177, -0.8) projected
  line L17 (-8.3177, -0.8) -> (-5.0268, -0.8)
  line L18 (-5.0268, -0.8) -> (-3.3813, -3.65)
  line L19 (-3.3813, -3.65) -> (-5.0268, -6.5)
  line L20 (-5.0268, -6.5) -> (-8.3177, -6.5)
  line L21 (-8.3177, -6.5) -> (-9.9631, -3.65)
  line L22 (-9.9631, -3.65) -> (-8.3177, -0.8)
  line L23 (0, 5.7) -> (9.4914, 5.7)
  line L24 (9.4914, 5.7) -> (9.4914, 0)
  line L25 (9.4914, 0) -> (0, 0)
  line L26 (0, 0) -> (0, 5.7)
  line L27 (0, -6.5) -> (5.6801, -6.5)
  line L28 (5.6801, -6.5) -> (5.6801, -0.8)
  line L29 (5.6801, -0.8) -> (0, -0.8)
  line L30 (0, -0.8) -> (0, -6.5)
  line L31 (0, 0) -> (-1.7321, 0) projected
  line L32 (-1.7321, -0.8) -> (0, -0.8) projected
  point P0 (28.3278, -8.65)
  point P1 (-5.0268, -0.8)
  point P2 (-5.0268, -6.5)
  point P3 (-5.0268, 5.7)
  point P4 (-5.0268, 0)
  constraints: 40 end point, 4 parallel, 2 coincident, 2 collinear, 2 horizontal, 2 perpendicular, 26 other
extrude "押し出し26" cut sketch "スケッチ29" against normal blind 3 contours L23 L24 L25 L0 | L0 L4 L12 L11 L1 | L29 L28 L27 L5 | L5 L9 L19 L18 L6
sketch "スケッチ30" plane through (-61.9714, 0, -72.4893) normal (-0.8660254, 0, -0.5) x (-0.5, 0, 0.8660254)
  circle A0 centre (-3.2081, 11.5) radius 1.6 projected
  circle A1 centre (-3.2081, 5) radius 1.6 projected
  point P0 (31.7919, 0)
extrude "押し出し27" cut sketch "スケッチ30" against normal blind 15
sketch "スケッチ31" plane through (-35.7081, 0, -27) normal (0, -1, 0) x (1, 0, 0)
  circle A0 centre (-13.2794, -31.8969) radius 1.6 projected
  point P0 (35.7081, 27)
extrude "押し出し28" cut sketch "スケッチ31" against normal blind 15
ref_plane "作業平面7" through (-88.2346, 0, -27) normal (0.5, 0, 0.8660254) x (0, 1, 0)
mirror "ミラー6" about plane through (-88.2346, 0, -27) normal (0.5, 0, 0.8660254) of "押し出し26", "押し出し27", "押し出し28"
sketch "スケッチ32" plane through (-35, 34.3, -57.735) normal (0, -1, 0) x (1, 0, 0)
  line L0 (0, 5.7446) -> (0, 0) projected
  line L1 (0, 5.7446) -> (-4.975, -2.8723) projected
  line L2 (0, 0) -> (-4.975, -2.8723) projected
  point P0 (35, 57.735)
extrude "押し出し29" cut sketch "スケッチ32" against normal through all
sketch "スケッチ33" plane through (-61.6173, 97, -73.1025) normal (0, 1, 0) x (1, 0, 0)
  line L0 (35.1173, -1.2224) -> (-12.5346, 26.2894) projected
  arc A0 (36.6173, -3.8205) -> (35.1173, -1.2224) centre (33.6173, -3.8205) ccw projected
  line L1 (36.6173, 0) -> (36.6173, -10.6025) projected
  line L2 (0, 0) -> (36.6173, 0) projected
  point P0 (61.6173, -73.1025)
  point P1 (33, 0)
extrude "押し出し30" cut sketch "スケッチ33" against normal through all
sketch "スケッチ34" plane through (-42.3476, 97, -38.5) normal (0, 1, 0) x (1, 0, 0)
  circle A0 centre (22.3476, 2.5) radius 5 projected
  line L0 (17.3476, -11.5) -> (17.3476, 0) projected
  line L1 (17.3476, -4.3426) -> (29.3476, -4.3426)
  line L2 (29.3476, -4.3426) -> (29.3476, -11.5)
  line L3 (29.3476, -11.5) -> (17.3476, -11.5)
  line L4 (17.3476, -11.5) -> (17.3476, -4.3426)
  line L5 (17.3476, -11.5) -> (6.6395, -11.5) projected
  circle A1 centre (25.3476, -7.9213) radius 1.6
  circle A2 centre (22.3476, 2.5) radius 6.8426
  line L6 (17.3476, -4.3426) -> (17.3476, 0)
  point P0 (42.3476, -38.5)
  point P1 (29.3476, -7.9213)
  point P2 (17.3476, -2.1713)
  point P3 (22.3476, -4.3426)
  point P4 (17.3476, -2.1713)
  dimension "d123" = 3.2
  dimension "d125" = 12
  dimension "d126" = 4
  constraints: 10 end point, 2 horizontal, 2 midpoint, 2 parallel, 1 centre point, 1 coincident, 1 collinear, 1 horizontal alignment, 1 perpendicular, 1 point on line, 1 vertical, 3 other
  measures "d123" diameter of A1
  measures "d125" distance of L2.end L3.end
  measures "d126" distance from line of L2 A1.centre
extrude "押し出し31" add sketch "スケッチ34" against normal up to surface (8 mm away) contours L0 L1 L2 L3 | L0 A2 L1
fillet "フィレット3" radius 3 2 edges at (-13, 93, -27) (-13, 93, -34.1574)
equation "\"d3\" = d2"
equation "\"d7\" = d4"
equation "\"BendRadius\" = Thickness"
equation "\"BendReliefWidth\" = Thickness"
equation "\"BendReliefDepth\" = 0.5 * Thickness"
equation "\"CornerReliefSize\" = 4 * Thickness"
equation "\"MinimumRemnant\" = 2 * Thickness"
equation "\"TransitionRadius\" = BendRadius"
equation "\"JacobiRadiusSize\" = BendRadius"
equation "\"GapSize\" = Thickness"
equation "\"Thickness\" = 1.5"
